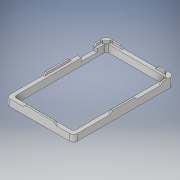
# Autodesk Inventor part: 3D_Printed_MALDI_Plate_Holder_V2
Saved by Autodesk Inventor 2019.3 (Build 233278000, 278)
## iProperties
Created: 2020-10-28
Part Number: 3D_Printed_MALDI_Plate_Holder_V2
Material: Generic
Document SubType Name: Modeling
Designer: schmidtg
Density: 1 g/cm^3
Appearance: Default
Author: schmidtg
Autodesk Inventor part; units mm, degrees
ref_plane "YZ Plane" through (0, 0, 0) normal (1, 0, 0) x (0, 1, 0)
ref_plane "XZ Plane" through (0, 0, 0) normal (0, 1, 0) x (-1, 0, 0)
ref_plane "XY Plane" through (0, 0, 0) normal (0, 0, 1) x (1, 0, 0)
sketch "Sketch1" plane through (0, 0, 0) normal (0, 1, 0) x (-1, 0, 0)
  line L0 (-5, 0) -> (-81, 0)
  line L1 (-86, 5) -> (-86, 122.95)
  line L2 (-81, 127.95) -> (-5, 127.95)
  line L3 (0, 122.95) -> (0, 5)
  arc A0 (0, 122.95) -> (-5, 127.95) centre (-5, 122.95) ccw
  arc A1 (-81, 127.95) -> (-86, 122.95) centre (-81, 122.95) ccw
  arc A2 (-86, 5) -> (-81, 0) centre (-81, 5) ccw
  arc A3 (-5, 0) -> (0, 5) centre (-5, 5) ccw
  point P0 (0, 0)
  point P1 (-86, 127.95)
  point P2 (-86, 0)
  point P3 (0, 127.95)
  dimension "d0" = 86
  dimension "d1" = 127.95
  dimension "d2" = 5
  constraints: 8 end point, 8 point on circle, 8 point on line, 8 tangent, 4 centre point, 3 equal radius, 2 parallel, 1 horizontal, 1 perpendicular
  measures "d0" distance of point (-86, 127.95) point (0, 127.95)
  measures "d1" distance of point (-86, 0) point (-86, 127.95)
  measures "d2" radius of A0
extrude "Extrusion1" add sketch "Sketch1" along normal blind 12
sketch "Sketch2" plane through (0, 12, 0) normal (0, 1, 0) x (1, 0, 0)
  line L0 (8.45, -2.025) -> (77.55, -2.025)
  line L1 (84.05, -8.525) -> (84.05, -125.925)
  line L2 (84.05, -125.925) -> (1.95, -125.925)
  line L3 (1.95, -125.925) -> (1.95, -8.525)
  line L4 (0, -5) -> (0, -122.95) projected
  line L5 (81, 0) -> (5, 0) projected
  line L6 (1.95, -8.525) -> (8.45, -2.025)
  line L7 (77.55, -2.025) -> (84.05, -8.525)
  circle A0 centre (1.95, -8.525) radius 1
  circle A1 centre (8.45, -2.025) radius 1
  circle A2 centre (77.55, -2.025) radius 1
  circle A3 centre (84.05, -8.525) radius 1
  line L8 (1.95, -125.925) -> (0, -125.925)
  line L9 (0, -125.925) -> (0, -80.925)
  line L10 (0, -80.925) -> (1.95, -80.925)
  line L11 (1.95, -80.925) -> (1.95, -125.925)
  line L12 (5, -127.95) -> (81, -127.95) projected
  line L13 (1.95, -125.925) -> (21.95, -125.925)
  line L14 (21.95, -125.925) -> (21.95, -127.95)
  line L15 (21.95, -127.95) -> (1.95, -127.95)
  line L16 (1.95, -127.95) -> (1.95, -125.925)
  line L17 (1.95, -125.925) -> (0, -125.925)
  line L18 (0, -125.925) -> (0, -127.95)
  line L19 (0, -127.95) -> (1.95, -127.95)
  line L20 (1.95, -127.95) -> (1.95, -125.925)
  line L21 (84.05, -125.925) -> (64.05, -125.925)
  line L22 (64.05, -125.925) -> (64.05, -127.95)
  line L23 (64.05, -127.95) -> (84.05, -127.95)
  line L24 (84.05, -127.95) -> (84.05, -125.925)
  line L25 (86, -122.95) -> (86, -5) projected
  line L26 (84.05, -125.925) -> (86, -125.925)
  line L27 (86, -125.925) -> (86, -80.925)
  line L28 (86, -80.925) -> (84.05, -80.925)
  line L29 (84.05, -80.925) -> (84.05, -125.925)
  line L30 (84.05, -125.925) -> (86, -125.925)
  line L31 (86, -125.925) -> (86, -127.95)
  line L32 (86, -127.95) -> (84.05, -127.95)
  line L33 (84.05, -127.95) -> (84.05, -125.925)
  line L34 (1.95, -17.025) -> (0, -17.025)
  line L35 (0, -17.025) -> (0, -47.025)
  line L36 (0, -47.025) -> (1.95, -47.025)
  line L37 (1.95, -47.025) -> (1.95, -17.025)
  line L38 (84.05, -47.025) -> (86, -47.025)
  line L39 (86, -47.025) -> (86, -17.025)
  line L40 (86, -17.025) -> (84.05, -17.025)
  line L41 (84.05, -17.025) -> (84.05, -47.025)
  line L42 (21.95, -2.025) -> (64.05, -2.025)
  line L43 (64.05, -2.025) -> (64.05, 0)
  line L44 (64.05, 0) -> (21.95, 0)
  line L45 (21.95, 0) -> (21.95, -2.025)
  point P0 (0, 0)
  point P1 (1.95, -2.025)
  point P2 (84.05, -2.025)
  point P3 (1.95, -125.925)
  point P4 (1.95, -8.525)
  point P5 (8.45, -2.025)
  point P6 (84.05, -8.525)
  dimension "d13" = 0
  dimension "d5" = 123.9
  dimension "d6" = 82.1
  dimension "d7" = 1.95
  dimension "d8" = 2.025
  dimension "d9" = 6.5
  dimension "d10" = 6.5
  dimension "d11" = 6.5
  dimension "d12" = 6.5
  dimension "d22" = 2
  dimension "d23" = 2
  dimension "d24" = 2
  dimension "d25" = 2
  dimension "d54" = 45
  dimension "d55" = 20
  dimension "d56" = 20
  dimension "d57" = 45
  dimension "d58" = 45
  dimension "d59" = 30
  dimension "d60" = 30
  dimension "d61" = 20
  dimension "d62" = 20
  constraints: 84 end point, 29 point on line, 20 parallel, 14 horizontal, 10 perpendicular, 4 centre point, 4 coincident, 4 vertical, 28 other
  measures "d5" distance of point (1.95, -125.925) point (1.95, -2.025)
  measures "d6" distance of point (1.95, -2.025) point (84.05, -2.025)
  measures "d7" distance between parallel lines of L4 L3
  measures "d8" distance between parallel lines of L5 L0
  measures "d9" distance of point (1.95, -8.525) point (1.95, -2.025)
  measures "d10" distance of point (8.45, -2.025) point (1.95, -2.025)
  measures "d11" distance of point (77.55, -2.025) point (84.05, -2.025)
  measures "d12" distance of point (84.05, -8.525) point (84.05, -2.025)
  measures "d22" diameter of A0
  measures "d23" diameter of A1
  measures "d24" diameter of A2
  measures "d25" diameter of A3
  measures "d54" distance of L8.end L9.end
  measures "d55" distance of L14.end L15.end
  measures "d56" distance of L23.end L22.end
  measures "d57" distance of L27.end L26.end
  measures "d58" distance between parallel lines of L36 L0
  measures "d59" distance from line of L36.end L34
  measures "d60" distance between parallel lines of L38 L40
  measures "d61" distance between parallel lines of L41 L43
  measures "d62" distance between parallel lines of L3 L45
extrude "Extrusion2" cut sketch "Sketch2" against normal blind 2.9 contours L6 A1 L0 | L0 A1 L6 | L0 A2 L7 A3 L1 L2 L3 A0 L6 A1 | L45 L5 L43 L0 | A0 L3 L6 | L6 L3 A0 | A2 L7 L0 | L0 L7 A2 | L3 L36 L4 L34 | A3 L1 L7 | L7 L1 A3 | L3 L8 L9 L4 L10 | L16 L19 L18 L8 | L2 L14 L12 L15 L16 | L40 L25 L38 L1 | L2 L24 L23 L12 L22 | L28 L25 L27 L26 L1 | L26 L31 L32 L24
fillet "Fillet1" radius 0.5 8 edges at (84.05, 10.55, 9.525) (83.3429, 10.55, 7.8179) (78.2571, 10.55, 2.7321) (76.55, 10.55, 2.025) (1.95, 10.55, 9.525) (2.6571, 10.55, 7.8179) (7.7429, 10.55, 2.7321) (9.45, 10.55, 2.025)
sketch "Sketch4" plane through (0, 9.1, 0) normal (0, 1, 0) x (1, 0, 0)
  line L0 (81, 0) -> (5, 0) projected
  line L1 (0, -37.025) -> (12, -37.025)
  line L2 (12, -37.025) -> (12, -17.025)
  line L3 (12, -17.025) -> (0, -17.025)
  line L4 (0, -17.025) -> (0, -37.025)
  line L5 (0, -17.025) -> (1.95, -17.025) projected
  point P0 (0, 0)
  dimension "d71" = 12
  dimension "d72" = 20
  dimension "d74" = 0
  constraints: 8 end point, 2 parallel, 1 horizontal, 1 perpendicular
  measures "d71" distance of L2.end L3.end
  measures "d72" distance of L1.end L2.end
  measures "d74" distance between parallel lines of L5 L3
extrude "Extrusion4" cut sketch "Sketch4" against normal blind 4.1
chamfer "Chamfer4" distance 0.5 distance2 0.5 8 edges at (0, 0, 63.975) (1.4645, 0, 126.4855) (43, 0, 127.95) (84.5355, 0, 126.4855) (86, 0, 63.975) (84.5355, 0, 1.4645) (43, 0, 0) (1.4645, 0, 1.4645) measured on face at (84.182, 0, 1.818) measured on face at (0, 0.5, 63.975) measured on face at (43, 0, 0.5) measured on face at (1.818, 0, 1.818) measured on face at (1.818, 0, 126.132) measured on face at (84.182, 0, 126.132) measured on face at (43, 0, 127.45) measured on face at (85.5, 0, 63.975)
sketch "Sketch5" plane through (0, 0, 0) normal (0, -1, 0) x (1, 0, 0)
  line L0 (78, 122.95) -> (8, 122.95)
  line L1 (5, 119.95) -> (5, 8)
  line L2 (8, 5) -> (78, 5)
  line L3 (81, 8) -> (81, 119.95)
  line L4 (86, 5) -> (86, 122.95) projected
  line L5 (81, 127.95) -> (5, 127.95) projected
  line L6 (0, 122.95) -> (0, 5) projected
  line L7 (5, 0) -> (81, 0) projected
  arc A0 (81, 119.95) -> (78, 122.95) centre (78, 119.95) ccw
  arc A1 (8, 122.95) -> (5, 119.95) centre (8, 119.95) ccw
  arc A2 (5, 8) -> (8, 5) centre (8, 8) ccw
  arc A3 (78, 5) -> (81, 8) centre (78, 8) ccw
  point P0 (0, 0)
  dimension "d47" = 5
  dimension "d48" = 5
  dimension "d49" = 5
  dimension "d50" = 5
  dimension "d51" = 3
  constraints: 8 end point, 8 point on circle, 8 tangent, 4 centre point, 3 equal radius, 2 parallel, 1 horizontal, 1 perpendicular
  measures "d47" distance between parallel lines of L4 L3
  measures "d48" distance between parallel lines of L5 L0
  measures "d49" distance between parallel lines of L1 L6
  measures "d50" distance between parallel lines of L7 L2
  measures "d51" radius of A0
extrude "Extrusion5" cut sketch "Sketch5" against normal blind 12
chamfer "Chamfer5" distance 2.9 angle 45 10 edges at (0.975, 12, 80.925) (0.975, 12, 47.025) (0.975, 12, 17.025) (21.95, 12, 1.0125) (64.05, 12, 1.0125) (85.025, 12, 17.025) (85.025, 12, 47.025) (85.025, 12, 80.925) (64.05, 12, 126.9375) (21.95, 12, 126.9375)
equation "\"d7\" = -0.5 * d6 + 0.5 * d0"
equation "\"d8\" = -0.5 * d5 + 0.5 * d1"
equation "\"d10\" = d9"
equation "\"d11\" = d9"
equation "\"d12\" = d11"
equation "\"d48\" = d47"
equation "\"d49\" = d47"
equation "\"d50\" = d47"
body "Solid1"
